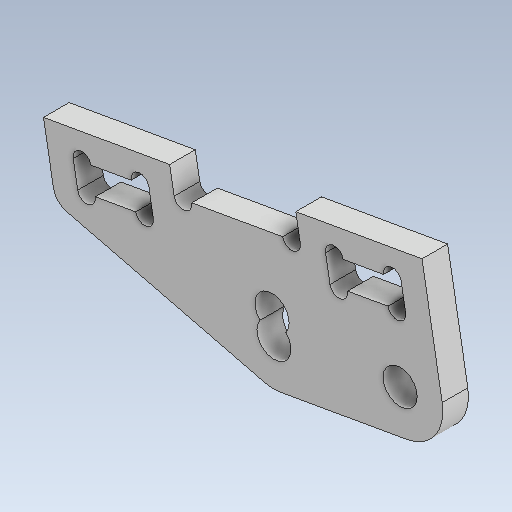
# Autodesk Inventor part: シールド根本
Saved by Autodesk Inventor 2020 (Build 240168000, 168)
## iProperties
Created: 2020-02-05
Part Number: シールド根本
Material: 一般
Document SubType Name: Modeling
Designer: tanjihayato
Density: 1 g/cm^3
Appearance: 既定
Mass: 1.66025 g
Surface Area: 17.4642 cm^2
Volume: 1.66025 cm^3
Author: tanjihayato
Autodesk Inventor part; units mm, degrees
ref_plane "YZ Plane" through (0, 0, 0) normal (1, 0, 0) x (0, 1, 0)
ref_plane "XZ Plane" through (0, 0, 0) normal (0, 1, 0) x (-1, 0, 0)
ref_plane "XY Plane" through (0, 0, 0) normal (0, 0, 1) x (1, 0, 0)
sketch "スケッチ1" plane through (0, 0, 0) normal (0, 0, 1) x (1, 0, 0)
  circle A0 centre (0, 0) radius 2
  circle A1 centre (-15, 0) radius 2
  line L0 (-41.2338, 3.4977) -> (3.0825, 11.3119)
  line L1 (-18.0894, 0) -> (0, 0)
  line L2 (3.0825, 11.3119) -> (2.5616, 14.2663)
  line L3 (2.5616, 14.2663) -> (-12.2105, 11.6616)
  line L4 (-12.2105, 11.6616) -> (-11.6896, 8.7071)
  line L5 (-26.4617, 6.1024) -> (-26.9826, 9.0568)
  line L6 (-26.9826, 9.0568) -> (-41.7547, 6.4521)
  line L7 (-41.7547, 6.4521) -> (-41.2338, 3.4977)
  line L8 (-41.2338, 3.4977) -> (-40.3656, -1.4264)
  line L9 (-40.3656, -1.4264) -> (-15.9724, -7.4585)
  arc A2 (0.8682, -4.924) -> (4.924, 0.8682) centre (0, 0) ccw
  line L10 (-13.9039, -7.5288) -> (0.8682, -4.924)
  line L11 (3.0825, 11.3119) -> (4.924, 0.8682)
  line L12 (-38.2794, 4.0186) -> (-37.7584, 1.0642)
  line L13 (-37.7584, 1.0642) -> (-28.8952, 2.627)
  line L14 (-28.8952, 2.627) -> (-29.4161, 5.5815)
  line L15 (-8.7351, 9.2281) -> (-8.2142, 6.2737)
  line L16 (-8.2142, 6.2737) -> (0.6491, 7.8365)
  line L17 (0.6491, 7.8365) -> (0.1281, 10.7909)
  circle A3 centre (-37.2453, 4.201) radius 1.05
  circle A4 centre (-30.4502, 5.3991) radius 1.05
  circle A5 centre (-29.9292, 2.4447) radius 1.05
  circle A6 centre (-36.7244, 1.2465) radius 1.05
  circle A7 centre (-7.7011, 9.4104) radius 1.05
  circle A8 centre (-0.9059, 10.6086) radius 1.05
  circle A9 centre (-0.385, 7.6542) radius 1.05
  circle A10 centre (-7.1802, 6.456) radius 1.05
  circle A11 centre (-25.4276, 6.2847) radius 1.05
  circle A12 centre (-12.7236, 8.5248) radius 1.05
  arc A13 (-15.9724, -7.4585) -> (-13.9039, -7.5288) centre (-14.7721, -2.6047) ccw
  line L18 (-14.7721, -2.6047) -> (0, 0)
  circle A14 centre (-14.7721, -2.6047) radius 2
  point P0 (-11.6896, 8.7071)
  point P1 (-13.7577, 8.3425)
  point P2 (-24.3936, 6.4671)
  point P3 (-26.4617, 6.1024)
  point P4 (-6.667, 9.5927)
  point P5 (-1.94, 10.4262)
  point P6 (0.1281, 10.7909)
  point P7 (-1.419, 7.4718)
  point P8 (-6.1461, 6.6383)
  point P9 (-8.2142, 6.2737)
  point P10 (-29.4161, 5.5815)
  point P11 (-28.8952, 2.627)
  point P12 (-30.9633, 2.2624)
  point P13 (-35.6903, 1.4289)
  point P14 (-37.7584, 1.0642)
  point P15 (-38.2794, 4.0186)
  point P16 (-36.2113, 4.3833)
  point P17 (-31.4842, 5.2168)
  point P18 (-16.3939, -1.4343)
  point P19 (-13.3783, -1.1704)
  dimension "d0" = 4
  dimension "d1" = 4
  dimension "d2" = 15
  dimension "d4" = 10
  dimension "d5" = 3
  dimension "d6" = 15
  dimension "d7" = 3
  dimension "d8" = 15
  dimension "d9" = 10
  dimension "d10" = 3
  dimension "d11" = 9
  dimension "d12" = 3
  dimension "d13" = 9
  dimension "d14" = 3
  dimension "d15" = 3
  dimension "d16" = 5
  dimension "d19" = 15
  dimension "d20" = 2.1
  dimension "d21" = 2.1
  dimension "d22" = 2.1
  dimension "d23" = 2.1
  dimension "d24" = 2.1
  dimension "d25" = 2.1
  dimension "d26" = 2.1
  dimension "d27" = 2.1
  dimension "d28" = 2.1
  dimension "d29" = 2.1
  dimension "d33" = 5
  dimension "d34" = 15
  dimension "d35" = 10
  dimension "d36" = 4
  dimension "d37" = 8
  constraints: 36 end point, 15 centre point, 14 tangent, 5 point on line, 4 point on circle, 3 coincident, 3 perpendicular, 2 collinear, 1 horizontal, 1 horizontal alignment, 1 parallel, 22 other
  measures "d0" diameter of A0
  measures "d1" diameter of A1
  measures "d2" distance of point (0, 0) A1.centre
  measures "d5" distance of L2.start L2.end
  measures "d6" distance of L2.end L3.end
  measures "d7" distance of L5.start L5.end
  measures "d8" distance of L5.end L6.end
  measures "d9" diameter of A2
  measures "d10" distance of L12.start L12.end
  measures "d11" distance of L12.end L13.end
  measures "d12" distance of L15.start L15.end
  measures "d13" distance of L15.end L16.end
  measures "d14" distance between parallel lines of L2 L17
  measures "d15" distance between parallel lines of L7 L12
  measures "d16" distance of L7.end L8.end
  measures "d19" distance between parallel lines of L5 L4
  measures "d20" diameter of A3
  measures "d21" diameter of A4
  measures "d22" diameter of A5
  measures "d23" diameter of A6
  measures "d24" diameter of A7
  measures "d25" diameter of A8
  measures "d26" diameter of A9
  measures "d27" diameter of A10
  measures "d28" diameter of A11
  measures "d29" diameter of A12
  measures "d33" radius of A13
  measures "d34" distance of L18.start L18.end
  measures "d35" angle of L18 L1
  measures "d36" diameter of A14
extrude "押し出し1" add sketch "スケッチ1" along normal blind 3 contours A0 L18 A14 A1 L1 | L7 L6 L5 L0 A4 A3 | L0 L12 A6 L13 A5 L14 A11 A12 L15 A10 L16 A9 L17 L11 A2 L10 A13 L9 L8 | L4 L3 L2 L0 A8 A7
fillet "フィレット1" radius 2 1 edges at (-40.3656, -1.4264, 1.5)
